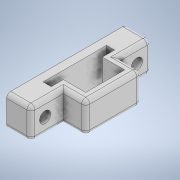
# Autodesk Inventor part: actuator_mounting
Saved by Autodesk Inventor 2021 (Build 250183000, 183)
## iProperties
Created: 2021-04-15
Part Number: actuator_mounting
Material: Generic
Document SubType Name: Modeling
Designer: Charlie
Density: 1 g/cm^3
Appearance: Default
Author: Charlie
Autodesk Inventor part; units mm, degrees
ref_plane "YZ Plane" through (0, 0, 0) normal (1, 0, 0) x (0, 1, 0)
ref_plane "XZ Plane" through (0, 0, 0) normal (0, 1, 0) x (-1, 0, 0)
ref_plane "XY Plane" through (0, 0, 0) normal (0, 0, 1) x (1, 0, 0)
sketch "Sketch1" plane through (0, 0, 0) normal (0, 1, 0) x (-1, 0, 0)
  line L0 (3.5, 9.65) -> (-7.5, 9.65)
  line L1 (-7.5, 9.65) -> (-7.5, -9.65)
  line L2 (-7.5, -9.65) -> (3.5, -9.65)
  line L3 (7.5, -9.65) -> (7.5, 9.65)
  line L4 (7.5, 9.65) -> (-7.5, -9.65) construction
  line L5 (-7.5, 9.65) -> (7.5, -9.65) construction
  line L6 (3.5, 9.65) -> (3.5, 15.65)
  line L7 (3.5, 15.65) -> (7.5, 15.65)
  line L8 (7.5, 15.65) -> (7.5, 9.65)
  line L9 (-7.5, 0) -> (7.5, 0) construction
  line L10 (3.5, -9.65) -> (3.5, -15.65)
  line L11 (3.5, -15.65) -> (7.5, -15.65)
  line L12 (7.5, -15.65) -> (7.5, -9.65)
  line L13 (11.5, 9.65) -> (11.5, -9.65)
  line L14 (11.5, -9.65) -> (11.5, -19.65)
  line L15 (-0.5, -19.65) -> (-0.5, -13.65)
  line L16 (-0.5, -13.65) -> (-11.5, -13.65)
  line L17 (-11.5, -13.65) -> (-11.5, 13.65)
  line L18 (-11.5, 13.65) -> (-0.5, 13.65)
  line L19 (-0.5, 13.65) -> (-0.5, 19.65)
  line L20 (11.5, 19.65) -> (11.5, 9.65)
  line L21 (11.5, 19.65) -> (11.5, 29.65)
  line L22 (11.5, 29.65) -> (-0.5, 29.65)
  line L23 (-0.5, 29.65) -> (-0.5, 19.65)
  line L24 (11.5, -19.65) -> (11.5, -29.65)
  line L25 (11.5, -29.65) -> (-0.5, -29.65)
  line L26 (-0.5, -29.65) -> (-0.5, -19.65)
  point P0 (0, 0)
  dimension "d0" = 15
  dimension "d1" = 19.3
  dimension "d2" = 4
  dimension "d3" = 6
  dimension "d4" = 4
  dimension "d5" = 10
  constraints: 54 end point, 6 parallel, 5 symmetric about line, 4 midpoint, 4 perpendicular, 1 horizontal, 1 vertical, 5 other
  measures "d0" distance of L3.start L1.end
  measures "d1" distance of L1.end L0.end
  measures "d2" distance of L6.end L7.end
  measures "d3" distance of L0.start L6.end
  measures "d4" distance between parallel lines of L3 L13
  measures "d5" distance of L20.start L21.end
extrude "Extrusion1" add sketch "Sketch1" along normal blind 15
sketch "Sketch2" plane through (0.5, 0, 29.65) normal (1, 0, 0) x (0, 0, -1)
  line L0 (0, 0) -> (0, 15) construction
  line L1 (0, 7.5) -> (7, 7.5) construction
  circle A0 centre (7, 7.5) radius 2.75
  line L2 (29.65, 0) -> (29.65, 27.4912) construction
  line L3 (59.3, 7.5) -> (52.3, 7.5) construction
  circle A1 centre (52.3, 7.5) radius 2.75
  dimension "d8" = 7
  dimension "d9" = 5.5
  constraints: 6 end point, 3 symmetric about line, 2 centre point, 2 coincident, 1 horizontal, 1 midpoint, 1 vertical, 1 other
  measures "d8" distance of L1.start L1.end
  measures "d9" diameter of A0
extrude "Extrusion2" cut sketch "Sketch2" against normal blind 15
fillet "Fillet1" radius 2 18 edges at (11.5, 7.5, 13.65) (11.5, 15, 0) (6, 15, 13.65) (11.5, 0, 0) (11.5, 7.5, -13.65) (6, 0, -13.65) (6, 0, 13.65) (0.5, 15, 21.65) (0.5, 0, 21.65) (0.5, 7.5, 29.65) (0.5, 0, -21.65) (0.5, 7.5, -29.65) (0.5, 15, -21.65) (-5.5, 0, -29.65) (-5.5, 15, 29.65) (-5.5, 0, 29.65) (-5.5, 15, -29.65) (6, 15, -13.65)
body "Solid1"
